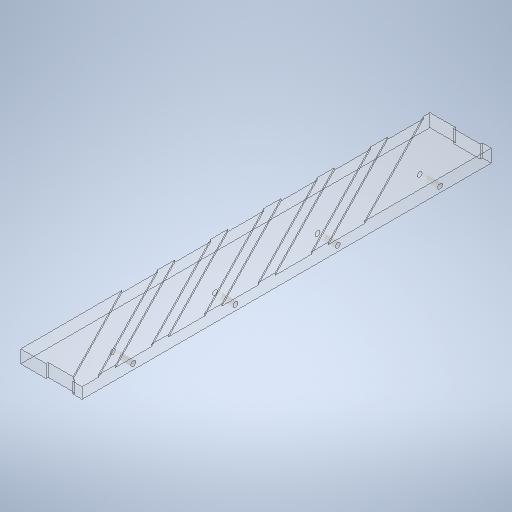
# Autodesk Inventor part: Module Cradle Left V1
Saved by Autodesk Inventor 2025 (Build 290162000, 162)
## iProperties
Created: 2024-03-20
Part Number: Module Cradle Left V1
Material: PMMA Plastic
Document SubType Name: Modeling
Designer: cfang
Density: 1.188 g/cm^3
Appearance: Polycarbonate - Clear
Author: cfang
Autodesk Inventor part; units mm, degrees
ref_plane "YZ Plane" through (0, 0, 0) normal (1, 0, 0) x (0, 1, 0)
ref_plane "XZ Plane" through (0, 0, 0) normal (0, 1, 0) x (-1, 0, 0)
ref_plane "XY Plane" through (0, 0, 0) normal (0, 0, 1) x (1, 0, 0)
sketch "Sketch3" plane through (0, 0, 0) normal (0, 1, 0) x (-1, 0, 0)
  line L0 (-15, -100) -> (15, -100)
  line L1 (15, -100) -> (15, 100)
  line L2 (15, 100) -> (-15, 100)
  line L3 (-15, 100) -> (-15, -100)
  line L4 (-15, -100) -> (15, 100) construction
  line L5 (15, -100) -> (-15, 100) construction
  point P0 (0, 0)
  dimension "d7" = 30
  dimension "d8" = 200
  constraints: 12 end point, 2 midpoint, 2 parallel, 1 horizontal, 1 perpendicular
  measures "d7" distance of L1.end L2.end
  measures "d8" distance of L0.end L1.end
extrude "Extrusion2" add sketch "Sketch3" along normal blind 6.35
sketch "Sketch4" plane through (0, 6.35, 0) normal (0, 1, 0) x (1, 0, 0)
  line L0 (-15, 100) -> (-15, -100) projected
  line L1 (-15, -50.7432) -> (15, -109.6215)
  line L2 (15, -100) -> (15, 100) projected
  line L3 (-15, -33.1217) -> (15, -92)
  line L4 (-15, -100) -> (15, -100) projected
  line L5 (-15, -24.7432) -> (15, -83.6215)
  line L6 (-15, -7.1217) -> (15, -66)
  line L7 (-15, 1.2568) -> (15, -57.6215)
  line L8 (-15, 18.8783) -> (15, -40)
  line L9 (-15, 27.2568) -> (15, -31.6215)
  line L10 (-15, 44.8783) -> (15, -14)
  line L11 (-15, 53.2568) -> (15, -5.6215)
  line L12 (-15, 70.8783) -> (15, 12)
  line L13 (-15, 79.2568) -> (15, 20.3785)
  line L14 (-15, 96.8783) -> (15, 38)
  point P0 (0, 0)
  point P1 (15, -50.386)
  point P2 (10.0976, -100)
  point P3 (15, 38)
  point P4 (-15, 96.8783)
  point P5 (15, 20.3785)
  point P6 (15, 12)
  point P7 (-15, 70.8783)
  point P8 (15, -5.6215)
  point P9 (15, -14)
  point P10 (-15, 44.8783)
  point P11 (15, -31.6215)
  point P12 (15, -40)
  point P13 (-15, 18.8783)
  point P14 (-15, 1.2568)
  point P15 (15, -57.6215)
  point P16 (15, -66)
  point P17 (-15, -7.1217)
  point P18 (15, -83.6215)
  dimension "d11" = 27
  dimension "d12" = 8
  dimension "d23" = 8
  dimension "d26" = 26
  constraints: 24 end point, 4 point on line, 1 parallel, 1 vertical, 30 other
  measures "d11" angle of L0 L1
  measures "d12" distance between parallel lines of L1 L3
  measures "d23" distance from line of L4 L3.end
  measures "d26" distance of L1.start L5.start
extrude "Extrusion3" cut sketch "Sketch4" against normal blind 1 contours L14 L2 L13 L0 | L12 L2 L11 L0 | L10 L2 L9 L0 | L8 L2 L7 L0 | L6 L2 L5 L0 | L3 L2 L4 L1 L0
sketch "Sketch7" plane through (-15, 0, 100) normal (0, 0, 1) x (1, 0, 0)
  line L0 (30, 6.35) -> (0, 6.35) projected
  line L1 (25.5, 0) -> (12.5, 0)
  line L2 (12.5, 0) -> (12.5, 6.35)
  line L3 (12.5, 6.35) -> (25.5, 6.35)
  line L4 (25.5, 6.35) -> (25.5, 0)
  line L5 (30, 0) -> (30, 5.35) projected
  point P0 (15, 0)
  point P1 (25.5, 6.35)
  dimension "d40" = 4.5
  dimension "d41" = 17.5
  constraints: 8 end point, 2 parallel, 1 horizontal, 1 perpendicular, 1 point on line
  measures "d40" distance between parallel lines of L4 L5
  measures "d41" distance between parallel lines of L2 L5
extrude "Extrusion5" cut sketch "Sketch7" against normal blind 1
sketch "Sketch8" plane through (15, 0, -100) normal (0, 0, -1) x (-1, 0, 0)
  line L0 (30, 6.35) -> (0, 6.35) projected
  line L1 (0, 0) -> (30, 0) projected
  line L2 (4.5, 6.35) -> (17.5, 6.35)
  line L3 (17.5, 6.35) -> (17.5, 0)
  line L4 (17.5, 0) -> (4.5, 0)
  line L5 (4.5, 0) -> (4.5, 6.35)
  line L6 (0, 0) -> (0, 6.35) projected
  point P0 (15, 0)
  point P1 (4.5, 0)
  dimension "d44" = 4.5
  dimension "d45" = 17.5
  constraints: 8 end point, 2 parallel, 2 point on line, 1 horizontal, 1 perpendicular
  measures "d44" distance between parallel lines of L5 L6
  measures "d45" distance between parallel lines of L3 L6
extrude "Extrusion6" cut sketch "Sketch8" against normal blind 1 contours L3 L1 L5 L0
sketch "Sketch9" plane through (15, 0, 100) normal (1, 0, 0) x (0, 0, -1)
  line L0 (0, 0) -> (200, 0) projected
  point P0 (100, 0)
  point P1 (25, 2.675)
  point P2 (75, 2.675)
  point P3 (125, 2.675)
  point P4 (175, 2.675)
  point P5 (100, 0)
  point P6 (100, 0)
  dimension "d48" = 2.675
  dimension "d49" = 25
  dimension "d50" = 50
  dimension "d51" = 25
  dimension "d52" = 50
  constraints: 3 horizontal alignment, 2 midpoint
  measures "d48" distance from line of L0 point (25, 2.675)
  measures "d49" horizontal distance of point (75, 2.675) point (100, 0)
  measures "d50" distance of point (25, 2.675) point (75, 2.675)
  measures "d51" horizontal distance of point (100, 0) point (125, 2.675)
  measures "d52" distance of point (125, 2.675) point (175, 2.675)
hole "Hole1" at (15, 2.675, 75) at (15, 2.675, 25) at (15, 2.675, -25) at (15, 2.675, -75) direction (-1, 0, 0) diameter 2.459 depth 10 tip angle 118 thread size "M3x0.5" class "6H" standard "ANSI Metric M Profile"
equation "\"d50\" = 2 * d49"
equation "\"d51\" = d49"
equation "\"d52\" = d50"
body "Solid2"
